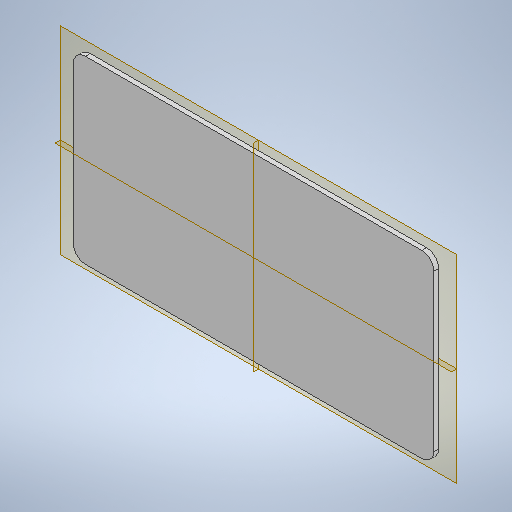
# Autodesk Inventor part: pernas_0001_00001
Saved by Autodesk Inventor 2025.2 (Build 292293000, 293)
## iProperties
Created: 2025-03-28
Part Number: pernas_0001_00001
Material: Generic
Document SubType Name: Modeling
Designer: kenne
Density: 1 g/cm^3
Appearance: Default
Author: kenne
Autodesk Inventor part; units mm, degrees
sketch "Sketch1" plane through (0, 0, 0) normal (0, 0, 1) x (1, 0, 0)
  line L0 (-750, -375) -> (750, -375)
  line L1 (750, -375) -> (750, 375)
  line L2 (750, 375) -> (-750, 375)
  line L3 (-750, 375) -> (-750, -375)
  line L4 (-750, -375) -> (750, 375) construction
  line L5 (750, -375) -> (-750, 375) construction
  point P0 (0, 0)
  dimension "d0" = 750
  dimension "d1" = 1500
  constraints: 12 end point, 2 midpoint, 2 parallel, 1 horizontal, 1 perpendicular
  measures "d0" distance between parallel lines of L2 L0
  measures "d1" distance between parallel lines of L1 L3
extrude "Extrusion1" add sketch "Sketch1" along normal blind 20
fillet "Fillet1" radius 50 4 edges at (750, 375, 10) (750, -375, 10) (-750, 375, 10) (-750, -375, 10)
body "Solid1"
